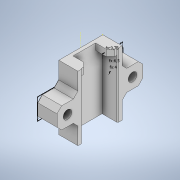
# Autodesk Inventor part: Profileend_fasterner
Saved by Autodesk Inventor 2021 (Build 250183000, 183)
## iProperties
Created: 2020-06-21
Part Number: Profileend_fasterner
Material: Generic
Document SubType Name: Modeling
Designer: oskar
Density: 1 g/cm^3
Appearance: Default
Author: oskar
## iProperties of the stored document _3DPrint.ipt
Created: 2020-06-21
Part Number: _3DPrint
Material: Generic
Document SubType Name: Modeling
Designer: oskar
Density: 1 g/cm^3
Appearance: Default
Author: oskar
Autodesk Inventor part; units mm, degrees
ref_plane "YZ Plane" through (0, 0, 0) normal (1, 0, 0) x (0, 1, 0)
ref_plane "XZ Plane" through (0, 0, 0) normal (0, 1, 0) x (-1, 0, 0)
ref_plane "XY Plane" through (0, 0, 0) normal (0, 0, 1) x (1, 0, 0)
sketch "Sketch1" plane through (0, 0, 0) normal (0, 1, 0) x (-1, 0, 0)
  line L0 (-3.65, 8.25) -> (3.65, 8.25)
  line L1 (3.65, 8.25) -> (3.65, -8.25)
  line L2 (3.65, -8.25) -> (-3.65, -8.25)
  line L3 (-3.65, -8.25) -> (-3.65, 8.25)
  line L4 (-3.65, 8.25) -> (3.65, -8.25) construction
  line L5 (3.65, 8.25) -> (-3.65, -8.25) construction
  line L6 (5.65, 10.25) -> (-3.65, 10.25)
  line L7 (-3.65, 10.25) -> (-3.65, -10.25)
  line L8 (-3.65, -10.25) -> (5.65, -10.25)
  line L9 (5.65, -10.25) -> (5.65, 10.25)
  line L10 (5.65, 10.25) -> (-3.65, -10.25) construction
  line L11 (-3.65, 10.25) -> (5.65, -10.25) construction
  line L12 (7.51, 0) -> (-5.51, 0) projected
  point P0 (0, 0)
  point P1 (0, 0)
  point P2 (0, 0)
  point P3 (1, 0)
  point P4 (1, 0)
  point P5 (-3.65, 8.25)
  point P6 (-3.65, -8.25)
  dimension "d4" = 7.3
  dimension "d5" = 16.5
  dimension "d6" = 2
  dimension "d7" = 2
  constraints: 24 end point, 7 midpoint, 4 parallel, 2 horizontal, 2 perpendicular, 1 coincident, 1 collinear
  measures "d4" distance of L1.end L2.end
  measures "d5" distance between parallel lines of L0 L2
  measures "d6" distance between parallel lines of L2 L8
  measures "d7" distance between parallel lines of L9 L1
extrude "Extrusion1" add sketch "Sketch1" along normal blind 30 contours L7 L6 L9 L12 L1 L0 | L12 L9 L8 L7 L2 L1
sketch "Sketch2" plane through (-5.65, 0, -10.25) normal (-1, 0, 0) x (0, 0, 1)
  point P0 (10.25, 0)
sketch "Sketch3" plane through (-5.65, 0, -10.25) normal (-1, 0, 0) x (0, 0, 1)
  line L0 (10.25, -6) -> (10.25, 36) construction
  line L1 (-9.75, 10.125) -> (0, 10.125)
  line L2 (0, 10.125) -> (0, 19.875)
  line L3 (0, 19.875) -> (-9.75, 19.875)
  line L4 (-9.75, 19.875) -> (-9.75, 10.125)
  line L5 (-9.75, 10.125) -> (0, 19.875) construction
  line L6 (0, 10.125) -> (-9.75, 19.875) construction
  line L7 (10.25, 15) -> (4.2192, 15) construction
  line L8 (0, 0) -> (0, 30) projected
  circle A0 centre (-4.875, 15) radius 2
  circle A1 centre (-4.875, 15) radius 3.25
  line L9 (30.25, 10.125) -> (20.5, 10.125)
  line L10 (20.5, 10.125) -> (20.5, 19.875)
  line L11 (20.5, 19.875) -> (30.25, 19.875)
  line L12 (30.25, 19.875) -> (30.25, 10.125)
  line L13 (30.25, 10.125) -> (20.5, 19.875) construction
  line L14 (20.5, 10.125) -> (30.25, 19.875) construction
  circle A2 centre (25.375, 15) radius 2
  circle A3 centre (25.375, 15) radius 3.25
  point P0 (10.25, 0)
  dimension "d10" = 9.75
  dimension "d11" = 4
  dimension "d14" = 6.5
  constraints: 26 end point, 8 symmetric about line, 6 midpoint, 4 centre point, 4 coincident, 2 horizontal, 2 parallel, 2 perpendicular, 2 point on line, 1 collinear, 2 other
  measures "d10" distance of L2.end L3.end
  measures "d11" diameter of A0
  measures "d14" diameter of A1
extrude "Extrusion2" add sketch "Sketch3" against normal up to surface (9.3 mm away) contours L4 L3 L2 L1 | A1 | L9 L10 L11 L12 | A3
extrude "Extrusion3" cut sketch "Sketch3" against normal blind 3.65 contours A1 | A3
chamfer "Chamfer1" distance 2.1667 angle 45 8 edges at (-1, 19.875, -10.25) (-1, 19.875, -20) (-1, 10.125, -20) (-1, 10.125, -10.25) (-1, 10.125, 10.25) (-1, 10.125, 20) (-1, 19.875, 20) (-1, 19.875, 10.25)
chamfer "Chamfer2" distance 0.4 angle 45 22 edges at (-5.65, 30, 0) (-5.65, 20.9583, -11.3333) (-5.65, 26.0208, -10.25) (-5.65, 19.875, -15.125) (-5.65, 18.7917, -18.9167) (-5.65, 15, -20) (-5.65, 11.2083, -18.9167) (-5.65, 10.125, -15.125) (-5.65, 15, -18.375) (-5.65, 9.0417, -11.3333) (-5.65, 3.9792, -10.25) (-5.65, 0, 0) (-5.65, 3.9792, 10.25) (-5.65, 9.0417, 11.3333) (-5.65, 26.0208, 10.25) (-5.65, 20.9583, 11.3333) (-5.65, 19.875, 15.125) (-5.65, 18.7917, 18.9167) (-5.65, 15, 20) (-5.65, 11.2083, 18.9167) (-5.65, 10.125, 15.125) (-5.65, 15, 11.875)
chamfer "Chamfer3" distance 0.4 angle 45 2 edges at (3.65, 15, -8.25) (3.65, 15, 8.25)
chamfer "Chamfer4" distance 1.25 angle 45 2 edges at (-2, 15, -18.375) (-2, 15, 11.875)
sketch "Sketch4" plane through (0, 30, 0) normal (0, 1, 0) x (1, 0, 0)
  line L0 (3.25, -8.25) -> (3.65, -8.65) projected
  line L1 (3.25, -8.25) -> (-3.65, -8.25) projected
  line L2 (-3.65, -8.25) -> (-3.65, 8.25) projected
  line L3 (-3.65, 8.25) -> (3.25, 8.25) projected
  line L4 (3.65, 8.65) -> (3.25, 8.25) projected
  line L5 (3.65, 8.65) -> (3.65, 10.25) projected
  line L6 (3.65, 10.25) -> (-5.25, 10.25) projected
  line L7 (-5.25, -10.25) -> (-5.25, 10.25) projected
  line L8 (-5.25, -10.25) -> (3.65, -10.25) projected
  line L9 (3.65, -10.25) -> (3.65, -8.65) projected
  line L10 (-3.65, -8.25) -> (-3.65, 8.25) projected
  line L11 (3.25, -8.25) -> (-3.65, -8.25) projected
  line L12 (-3.65, -5.25) -> (3.25, -5.25)
  line L13 (3.25, -5.25) -> (3.25, -8.25)
  line L14 (3.25, -8.25) -> (-3.65, -8.25)
  line L15 (-3.65, -8.25) -> (-3.65, -5.25)
  line L16 (-3.65, 8.25) -> (3.25, 8.25)
  line L17 (3.25, 8.25) -> (3.25, 5.25)
  line L18 (3.25, 5.25) -> (-3.65, 5.25)
  line L19 (-3.65, 5.25) -> (-3.65, 8.25)
  point P0 (0, 0)
  point P1 (-3.65, 5.25)
  point P2 (-3.65, 5.25)
  dimension "d29" = 3
  dimension "d30" = 3
  constraints: 16 end point, 4 parallel, 2 horizontal, 2 perpendicular, 2 point on line
  measures "d29" distance of L12.end L0.start
  measures "d30" distance of L16.end L17.end
extrude "Extrusion4" add sketch "Sketch4" against normal blind 3 contours L1 L2 L12 L13 | L2 L3 L17 L18
chamfer "Chamfer5" distance 2 angle 45 2 edges at (3.25, 28.5, -5.25) (3.25, 28.5, 5.25)
equation "\"d4\" = H_Profile"
equation "\"d5\" = W_Profile"
equation "\"d6\" = T_Wall"
equation "\"d7\" = T_Wall"
equation "\"d8\" = L_Profile"
equation "\"d10\" = 1.5 * D_Screwhead"
equation "\"d11\" = D_Screw"
equation "\"d14\" = D_Screwhead"
equation "\"d15\" = 0.5 * H_Profile"
equation "\"d17\" = 0.333333 * D_Screwhead"
equation "\"d26\" = -0.5 * D_Screw + 0.5 * D_Screwhead"
equation "\"d29\" = d30"
equation "\"d31\" = d30"
equation "\"W_Profile\" = 16.5"
equation "\"H_Profile\" = 7.3"
equation "\"L_Profile\" = 30"
equation "\"T_Wall\" = 2"
equation "\"D_Screwhead\" = 6.5"
equation "\"D_Screw\" = 4"
body "Solid1"
